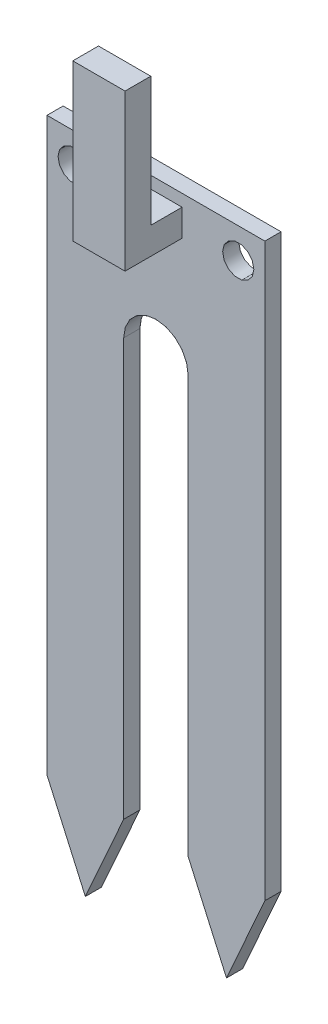
# Autodesk Inventor part: moist probe
Saved by Autodesk Inventor 2017 (Build 210142000, 142)
## iProperties
Created: 2017-04-29
Part Number: moist probe
Material: Generic
Document SubType Name: Modeling
Designer: X220T
Density: 1 g/cm^3
Appearance: Default
Author: X220T
Autodesk Inventor part; units mm, degrees
ref_plane "YZ Plane" through (0, 0, 0) normal (1, 0, 0) x (0, 1, 0)
ref_plane "XZ Plane" through (0, 0, 0) normal (0, 1, 0) x (-1, 0, 0)
ref_plane "XY Plane" through (0, 0, 0) normal (0, 0, 1) x (1, 0, 0)
sketch "Sketch1" plane through (0, 0, 0) normal (0, 0, 1) x (1, 0, 0)
  line L0 (-10.125, -30.55) -> (10.125, -30.55) construction
  line L1 (10.125, -30.55) -> (10.125, 30.55) construction
  line L2 (10.125, 30.55) -> (-10.125, 30.55)
  line L3 (-10.125, 30.55) -> (-10.125, -30.55) construction
  line L4 (-10.125, -30.55) -> (10.125, 30.55) construction
  line L5 (10.125, -30.55) -> (-10.125, 30.55) construction
  line L6 (-10.125, 30.55) -> (-10.125, -22.55)
  line L7 (-10.125, -22.55) -> (-6.56, -30.55)
  line L8 (-6.56, -30.55) -> (-2.995, -22.55)
  line L9 (-2.995, -22.55) -> (-2.995, 16.2)
  arc A0 (2.995, 16.2) -> (-2.995, 16.2) centre (0, 16.2) ccw
  line L10 (0, 0) -> (0, 8.9972) construction
  line L11 (10.125, 30.55) -> (10.125, -30.55) construction
  line L12 (10.125, 30.55) -> (10.125, -22.55)
  line L13 (10.125, -22.55) -> (6.56, -30.55)
  line L14 (6.56, -30.55) -> (2.995, -22.55)
  line L15 (2.995, -22.55) -> (2.995, 16.2)
  dimension "d0" = 20.25
  dimension "d1" = 61.1
  dimension "d2" = 8
  dimension "d3" = 3.565
  dimension "d4" = 14.35
  constraints: 32 end point, 4 symmetric about line, 3 point on line, 2 midpoint, 2 parallel, 2 point on circle, 2 vertical, 1 centre point, 1 equal length, 1 horizontal, 1 horizontal alignment, 1 perpendicular, 1 tangent, 1 vertical alignment
  measures "d0" distance of L2.end L1.end
  measures "d1" distance of L1.end L0.end
  measures "d2" vertical distance of L6.end L7.end
  measures "d3" distance from line of L3 L7.end
  measures "d4" distance from line of A0.centre L2
extrude "Extrusion1" add sketch "Sketch1" along normal blind 1.5
sketch "Sketch2" plane through (0, 0, 1.5) normal (0, 0, 1) x (1, 0, 0)
  line L0 (-2.43, 29.43) -> (2.43, 29.43)
  line L1 (2.43, 29.43) -> (2.43, 26.93)
  line L2 (2.43, 26.93) -> (-2.43, 26.93)
  line L3 (-2.43, 26.93) -> (-2.43, 29.43)
  line L4 (-2.43, 29.43) -> (2.43, 26.93) construction
  line L5 (2.43, 29.43) -> (-2.43, 26.93) construction
  line L6 (10.125, 30.55) -> (-10.125, 30.55) projected
  point P0 (0, 0)
  point P1 (0, 28.18)
  dimension "d7" = 4.86
  dimension "d8" = 2.5
  dimension "d9" = 1.12
  constraints: 12 end point, 2 midpoint, 2 parallel, 1 horizontal, 1 perpendicular, 1 vertical alignment
  measures "d7" distance of L1.end L2.end
  measures "d8" distance of L0.end L1.end
  measures "d9" distance between parallel lines of L6 L0
extrude "Extrusion2" add sketch "Sketch2" along normal blind 5.3
sketch "Sketch3" plane through (-2.43, 29.43, 1.5) normal (0, 1, 0) x (1, 0, 0)
  line L0 (0, 0) -> (0, -5.3) projected
  line L1 (0, -5.3) -> (4.86, -5.3)
  line L2 (4.86, -5.3) -> (4.86, -2.91)
  line L3 (4.86, -2.91) -> (0, -2.91)
  line L4 (0, -2.91) -> (0, -5.3)
  line L5 (4.86, 0) -> (4.86, -5.3) projected
  point P0 (2.43, 1.5)
  dimension "d12" = 2.39
  constraints: 8 end point, 2 parallel, 1 collinear, 1 horizontal, 1 perpendicular
  measures "d12" distance between parallel lines of L1 L3
extrude "Extrusion3" add sketch "Sketch3" along normal blind 12
sketch "Sketch4" plane through (0, 0, 1.5) normal (0, 0, 1) x (1, 0, 0)
  line L0 (-7.65, 27.75) -> (7.65, 27.75) construction
  circle A0 centre (-7.65, 27.75) radius 1.45
  circle A1 centre (7.65, 27.75) radius 1.45
  line L1 (10.125, 30.55) -> (-10.125, 30.55) projected
  point P0 (0, 0)
  point P1 (0, 27.75)
  point P2 (-7.65, 29.2)
  point P3 (-6.2, 27.75)
  point P4 (6.2, 27.75)
  dimension "d15" = 2.9
  dimension "d16" = 12.4
  dimension "d17" = 1.35
  constraints: 2 coincident, 2 end point, 2 point on circle, 2 point on line, 2 vertical alignment, 1 centre point, 1 horizontal, 1 horizontal alignment, 1 midpoint, 3 other
  measures "d15" diameter of A0
  measures "d16" distance of A0.end point (6.2, 27.75)
  measures "d17" distance from line of L1 A0.start
extrude "Extrusion4" cut sketch "Sketch4" against normal through all
body "Solid1"
